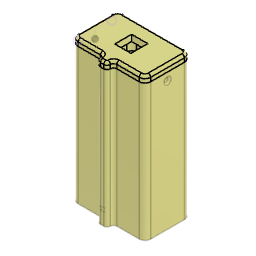
DelayPower Module Case (Autodesk Fusion 360 design; units mm, degrees)
Autodesk Fusion 360 part; units mm, degrees
sketch "Footprint" plane through (0, 0, 0) normal (0, 0, 1) x (1, 0, 0) in component "Case"
  line L0 (-12.76, 11.28) -> (12.76, 11.28)
  line L1 (15.18, 8.86) -> (15.18, -8.86)
  line L2 (12.76, -11.28) -> (-12.76, -11.28)
  line L3 (-15.18, -8.86) -> (-15.18, 8.86)
  arc A0 (-12.76, 11.28) -> (-15.18, 8.86) centre (-12.76, 8.86) ccw
  arc A1 (-15.18, -8.86) -> (-12.76, -11.28) centre (-12.76, -8.86) ccw
  arc A2 (12.76, -11.28) -> (15.18, -8.86) centre (12.76, -8.86) ccw
  arc A3 (15.18, 8.86) -> (12.76, 11.28) centre (12.76, 8.86) ccw
  line L4 (-7.205, 3.285) -> (-5.445, 3.285)
  line L5 (-5.445, 3.285) -> (-5.445, -3.285)
  line L6 (-5.445, -3.285) -> (-7.205, -3.285)
  line L7 (-7.205, -3.285) -> (-7.205, 3.285)
  line L8 (0, -11.28) -> (0, 11.28) construction
  line L9 (0, 0) -> (-5.445, 0) construction
  line L10 (7.205, -3.285) -> (7.205, 3.285)
  line L11 (5.445, 3.285) -> (5.445, -3.285)
  line L12 (7.205, 3.285) -> (5.445, 3.285)
  line L13 (5.445, -3.285) -> (7.205, -3.285)
  arc A4 (-18.6, 13.78) -> (-22.1, 10.28) centre (-18.6, 10.28) ccw
  line L14 (-22.1, -10.28) -> (-22.1, 10.28)
  arc A5 (-22.1, -10.28) -> (-18.6, -13.78) centre (-18.6, -10.28) ccw
  line L15 (-5, -13.78) -> (-18.6, -13.78)
  arc A6 (18.6, -13.78) -> (22.1, -10.28) centre (18.6, -10.28) ccw
  line L16 (22.1, 10.28) -> (22.1, -10.28)
  arc A7 (22.1, 10.28) -> (18.6, 13.78) centre (18.6, 10.28) ccw
  line L17 (-18.6, 13.78) -> (18.6, 13.78)
  line L18 (3, -15.7772) -> (3, -15.7772)
  line L19 (1, -17.78) -> (-1, -17.78)
  line L20 (-3, -15.7772) -> (-3, -15.7772)
  line L21 (1.8, -13.78) -> (1.8, -16.58)
  line L22 (1.8, -16.58) -> (-1.8, -16.58)
  line L23 (-1.8, -16.58) -> (-1.8, -13.78)
  arc A8 (-3, -15.7772) -> (-5, -13.78) centre (-5, -15.78) ccw
  line L24 (18.6, -13.78) -> (5, -13.78)
  arc A9 (5, -13.78) -> (3, -15.7772) centre (5, -15.78) ccw
  line L25 (1.8, -13.78) -> (-1.8, -13.78)
  line L26 (0, -11.28) -> (0, -13.78) construction
  arc A10 (-3, -15.7772) -> (-1, -17.78) centre (-1, -15.78) ccw
  arc A11 (1, -17.78) -> (3, -15.7772) centre (1, -15.78) ccw
  line L27 (19.6, -11.28) -> (19.6, 11.28)
  line L28 (-19.6, 11.28) -> (-19.6, -11.28)
  line L29 (-12.76, -11.28) -> (-19.6, -11.28)
  line L30 (12.76, -11.28) -> (19.6, -11.28)
  line L31 (12.76, 11.28) -> (19.6, 11.28)
  line L32 (-12.76, 11.28) -> (-19.6, 11.28)
  point P0 (5.445, 0)
  dimension "d1" = 2.42
  dimension "d2" = 2.42
  dimension "d3" = 2.42
  dimension "d4" = 2.42
  dimension "d5" = 30.36
  dimension "d6" = 22.56
  dimension "d7" = 1.76
  dimension "d8" = 6.57
  dimension "d9" = 5.445
  dimension "d15" = 1.2
  dimension "d16" = 2
  dimension "d17" = 2
  dimension "d23" = 2
  dimension "d24" = 2
  dimension "d25" = 1.2
  dimension "d26" = 1.2
  dimension "d27" = 4
  dimension "d28" = 6
  dimension "d76" = 3.5
  dimension "d77" = 3.5
  dimension "d78" = 3.5
  dimension "d79" = 3.5
  dimension "d80" = 39.2
  dimension "d81" = 2.5
  dimension "d82" = 2.5
  dimension "d83" = 2.5
  constraint horizontal L0
  constraint vertical L1
  constraint horizontal L2
  constraint vertical L3
  constraint tangent L0 A0
  constraint tangent L3 A0
  constraint tangent L2 A1
  constraint tangent L3 A1
  constraint tangent L1 A2
  constraint tangent L2 A2
  constraint tangent L0 A3
  constraint tangent L1 A3
  constraint horizontal L4
  constraint vertical L5
  constraint horizontal L6
  constraint vertical L7
  constraint midpoint L2 L8.start
  constraint midpoint L0 L8.end
  constraint midpoint L9.start L8
  constraint coincident L9.start origin
  constraint midpoint L5 L9.end
  constraint horizontal L9
  constraint symmetric L4.start L8 L10.end
  constraint symmetric L4.end L8 L11.start
  constraint symmetric L5.end L8 L11.end
  constraint symmetric L6.end L8 L10.start
  constraint symmetric L8 L9.end P0
  constraint horizontal L19
  constraint coincident L15 L21.start
  constraint perpendicular L15 L21
  constraint coincident L15 L23.end
  constraint perpendicular L22 L23
  constraint parallel L3 L14
  constraint parallel L2 L15
  constraint parallel L1 L16
  constraint parallel L0 L17
  constraint tangent A4 L17
  constraint tangent A4 L14
  constraint tangent A7 L17
  constraint tangent L14 A5
  constraint tangent A5 L15
  constraint tangent L16 A7
  constraint tangent L15 A6
  constraint tangent A6 L16
  constraint coincident A6.start L15
  constraint tangent L15 A8
  constraint tangent A6 L24
  constraint tangent L24 A9
  constraint midpoint L25 L26.end
  constraint perpendicular L25 L26
  constraint tangent L19 A10
  constraint tangent L19 A11
  constraint equal L15 L24
  constraint vertical L27
  constraint vertical L28
  constraint perpendicular L28 L29
  constraint perpendicular L27 L30
  constraint perpendicular L28 L32
  constraint perpendicular L27 L31
  constraint equal L29 L30
  measures "d1" radius of A0
  measures "d2" radius of A1
  measures "d3" radius of A2
  measures "d4" radius of A3
  measures "d5" distance of L1 L3
  measures "d6" distance of L0 L2
  measures "d7" distance of L4.start L4.end
  measures "d8" distance of L4.start L6.end
  measures "d9" distance of L9.start L9.end
  measures "d15" distance of L19 L22
  measures "d16" radius of A8
  measures "d17" radius of A9
  measures "d23" radius of A10
  measures "d24" radius of A11
  measures "d25" distance of L21 L18.start
  measures "d26" distance of L23 L20.start
  measures "d27" distance of L19 L24
  measures "d28" distance of L20.start L18.start
  measures "d76" radius of A5
  measures "d77" radius of A6
  measures "d78" radius of A7
  measures "d79" radius of A4
  measures "d80" distance of L27 L28
  measures "d81" distance of L14 L28
  measures "d82" distance of L2 L15
  measures "d83" distance of L0 L17
extrude "Extrude1" add sketch "Footprint" along normal blind 1.1 contours L0 L1 L2 L3 A0 A1 A2 A3 | L3 A0 A1 L28 L29 L32 | L1 A2 A3 L27 L30 L31 | A4 L14 A5 L15 A6 L16 A7 L17 L19 A8 L24 A9 A10 A11 | L21 L22 L23 L25 makes body 1 in component "Case"
extrude "Extrude2" add sketch "Footprint" along normal blind 81.8 from surface at 1.1 contours A4 L14 A5 L15 A6 L16 A7 L17 L19 A8 L24 A9 A10 A11 bodies 1 in component "Case"
sketch "WireCutouts" plane through (0, -13.78, 0) normal (0, -1, 0) x (1, 0, 0) in component "Case"
  line L0 (-1.8, 1.1) -> (1.8, 1.1)
  line L1 (1.8, 1.1) -> (1.8, 82.9)
  line L2 (1.8, 82.9) -> (-1.8, 82.9)
  line L3 (-1.8, 82.9) -> (-1.8, 1.1)
  line L4 (1.8, 67.9) -> (-1.8, 67.9)
  line L5 (1.8, 10.1) -> (-1.8, 10.1)
  line L6 (1.8, 7.1) -> (-1.8, 7.1)
  dimension "d29" = 15
  dimension "d30" = 3
  dimension "d31" = 6
  constraint coincident L1 L4.start
  constraint coincident L3 L4.end
  constraint perpendicular L3 L4
  constraint coincident L1 L5.start
  constraint coincident L3 L5.end
  constraint perpendicular L3 L5
  constraint coincident L1 L6.start
  constraint coincident L3 L6.end
  constraint perpendicular L3 L6
  measures "d29" distance of L2 L4
  measures "d30" distance of L5 L6
  measures "d31" distance of L0 L6
extrude "Extrude3" cut sketch "WireCutouts" against normal up to surface (2.5 mm away) contours L1 L2 L3 L4 bodies 1 in component "Case"
extrude "Extrude4" cut sketch "WireCutouts" along normal up to surface (1.2 mm away) draft -25 from surface at 2.8 contours L1 L3 L5 L6 bodies 1 in component "Case"
chamfer "Chamfer1" distance 0.5 angle 45 4 edges at (0, -13.78, 67.9) (-1.8, -13.93, 82.9) (0, -16.58, 82.9) (1.8, -13.93, 82.9) on bodies 1 in component "Case"
sketch "Profile" plane through (0, 0, 0) normal (0, 0, 1) x (1, 0, 0) in component "Plug Retainer"
  line L0 (-19.6, 11.28) -> (-19.6, -11.28)
  line L1 (-12.76, 11.28) -> (-19.6, 11.28)
  line L2 (-12.76, 11.28) -> (12.76, 11.28)
  line L3 (12.76, 11.28) -> (19.6, 11.28)
  line L4 (19.6, -11.28) -> (19.6, 11.28)
  line L5 (12.76, -11.28) -> (19.6, -11.28)
  line L6 (12.76, -11.28) -> (-12.76, -11.28)
  line L7 (-12.76, -11.28) -> (-19.6, -11.28)
  line L8 (-12.76, -11.125) -> (-19.445, -11.125)
  line L9 (-19.445, 11.125) -> (-19.445, -11.125)
  line L10 (-12.76, 11.125) -> (-19.445, 11.125)
  line L11 (-12.76, 11.125) -> (12.76, 11.125)
  line L12 (12.76, 11.125) -> (19.445, 11.125)
  line L13 (19.445, -11.125) -> (19.445, 11.125)
  line L14 (12.76, -11.125) -> (19.445, -11.125)
  line L15 (12.76, -11.125) -> (-12.76, -11.125)
  line L16 (-12.76, 8.86) -> (12.76, 8.86)
  line L17 (12.76, 8.86) -> (12.76, -8.86)
  line L18 (12.76, -8.86) -> (-12.76, -8.86)
  line L19 (-12.76, -8.86) -> (-12.76, 8.86)
  line L20 (-17.6, 10.08) -> (17.6, 10.08)
  line L21 (17.6, 10.08) -> (17.6, -10.08)
  line L22 (17.6, -10.08) -> (-17.6, -10.08)
  line L23 (-17.6, -10.08) -> (-17.6, 10.08)
  point P0 (-12.76, 8.86)
  point P1 (-12.76, -8.86)
  point P2 (12.76, -8.86)
  point P3 (12.76, 8.86)
  dimension "d84" = 0.155
  dimension "d85" = 2
  dimension "d86" = 2
  dimension "d87" = 1.2
  dimension "d88" = 1.2
  constraint horizontal L16
  constraint vertical L17
  constraint horizontal L18
  constraint vertical L19
  constraint coincident P2 L17.end
  constraint coincident P0 L16.start
  constraint horizontal L20
  constraint vertical L21
  constraint horizontal L22
  constraint vertical L23
  measures "d85" distance of L4 L21
  measures "d86" distance of L0 L23
  measures "d87" distance of L6 L22
  measures "d88" distance of L2 L20
extrude "Extrude1'" add sketch "Profile" along normal blind 3 from surface at 4.9 separate body contours L8 L9 L10 L11 L12 L13 L14 L15 | L20 L21 L22 L23 makes body 2 in component "Plug Retainer"
extrude "Extrude3'" add sketch "Profile" along normal up to surface (67 mm away) from surface at 7.9 contours L8 L9 L10 L11 L12 L13 L14 L15 bodies 2 in component "Plug Retainer"
extrude "Extrude2'" cut sketch "WireCutouts" against normal up to surface (3.7 mm away) contours L1 L2 L3 L4 bodies 2 in component "Plug Retainer"
sketch "Footprint (2)" plane through (0, 0, 0) normal (0, 0, 1) x (1, 0, 0) in component "Lid"
  arc A0 (-3, -15.7772) -> (-5, -13.78) centre (-5, -15.78) ccw
  line L0 (-5, -13.78) -> (-18.6, -13.78)
  arc A1 (-22.1, -10.28) -> (-18.6, -13.78) centre (-18.6, -10.28) ccw
  line L1 (-22.1, -10.28) -> (-22.1, 10.28)
  arc A2 (-18.6, 13.78) -> (-22.1, 10.28) centre (-18.6, 10.28) ccw
  line L2 (-18.6, 13.78) -> (18.6, 13.78)
  arc A3 (22.1, 10.28) -> (18.6, 13.78) centre (18.6, 10.28) ccw
  arc A4 (18.6, -13.78) -> (22.1, -10.28) centre (18.6, -10.28) ccw
  line L3 (18.6, -13.78) -> (5, -13.78)
  arc A5 (5, -13.78) -> (3, -15.7772) centre (5, -15.78) ccw
  line L4 (22.1, 10.28) -> (22.1, -10.28)
  arc A6 (1, -17.78) -> (3, -15.7772) centre (1, -15.78) ccw
  arc A7 (-3, -15.7772) -> (-1, -17.78) centre (-1, -15.78) ccw
  line L5 (1, -17.78) -> (-1, -17.78)
  line L6 (-5.905, 9.105) -> (5.905, 9.105)
  line L7 (8.905, 6.105) -> (8.905, -6.105)
  line L8 (5.905, -9.105) -> (-5.905, -9.105)
  line L9 (-8.905, -6.105) -> (-8.905, 6.105)
  line L10 (15.025, 0) -> (8.905, 0) construction
  line L11 (0, 9.105) -> (0, 11.125) construction
  arc A8 (-5.905, 9.105) -> (-8.905, 6.105) centre (-5.905, 6.105) ccw
  arc A9 (-8.905, -6.105) -> (-5.905, -9.105) centre (-5.905, -6.105) ccw
  arc A10 (5.905, -9.105) -> (8.905, -6.105) centre (5.905, -6.105) ccw
  arc A11 (8.905, 6.105) -> (5.905, 9.105) centre (5.905, 6.105) ccw
  line L12 (-4.905, 5.105) -> (4.905, 5.105)
  line L13 (4.905, 5.105) -> (4.905, -5.105)
  line L14 (4.905, -5.105) -> (-4.905, -5.105)
  line L15 (-4.905, -5.105) -> (-4.905, 5.105)
  line L16 (8.905, 0) -> (4.905, 0) construction
  line L17 (0, 9.105) -> (0, 5.105) construction
  line L18 (-19.445, 11.125) -> (-19.445, -11.125)
  line L19 (-12.76, 11.125) -> (-19.445, 11.125)
  line L20 (-12.76, 11.125) -> (12.76, 11.125)
  line L21 (12.76, 11.125) -> (19.445, 11.125)
  line L22 (19.445, -11.125) -> (19.445, 11.125)
  line L23 (12.76, -11.125) -> (19.445, -11.125)
  line L24 (12.76, -11.125) -> (-12.76, -11.125)
  line L25 (-12.76, -11.125) -> (-19.445, -11.125)
  dimension "d14" = 1.2
  dimension "d71" = 3
  dimension "d72" = 9.81
  dimension "d73" = 10.21
  dimension "d74" = 4
  dimension "d75" = 4
  constraint horizontal L6
  constraint vertical L7
  constraint horizontal L8
  constraint vertical L9
  constraint vertical L11
  constraint horizontal L10
  constraint coincident L6 L11.start
  constraint tangent L6 A8
  constraint tangent L9 A8
  constraint tangent L8 A9
  constraint tangent L9 A9
  constraint equal A8 A9
  constraint coincident L7 L10.end
  constraint tangent L7 A10
  constraint tangent L8 A10
  constraint equal A8 A10
  constraint tangent L6 A11
  constraint tangent L7 A11
  constraint equal A8 A11
  constraint midpoint L7 L10.end
  constraint midpoint L6 L11.start
  constraint horizontal L12
  constraint vertical L13
  constraint horizontal L14
  constraint vertical L15
  constraint midpoint L13 L16.end
  constraint midpoint L12 L17.end
  constraint vertical L17
  constraint horizontal L16
  constraint midpoint L11.end L20
  measures "d71" radius of A8
  measures "d72" distance of L13.end L14.end
  measures "d73" distance of L12.end L13.end
  measures "d74" distance of L11.start L17.end
  measures "d75" distance of L9 L15
extrude "Extrude4'" add sketch "Footprint (2)" along normal up to surface (8 mm away) from surface at 75.055 separate body contours L18 L19 L20 L21 L22 L23 L24 L25 makes body 3 in component "Lid"
extrude "Extrude5" add sketch "Footprint (2)" along normal blind 3.8 from surface at 83.055 contours A0 L0 A1 L1 A2 L2 A3 A4 L3 A5 L4 A6 A7 L5 | L6 L7 L8 L9 A8 A9 A10 A11 | L18 L19 L20 L21 L22 L23 L24 L25 bodies 3 in component "Lid"
fillet "Fillet2" radius 1.5 14 edges at (3.5868, -14.3648, 86.855) (11.8, -13.78, 86.855) (21.0749, -12.7549, 86.855) (22.1, 0, 86.855) (21.0749, 12.7549, 86.855) (0, 13.78, 86.855) (-21.0749, 12.7549, 86.855) (-22.1, 0, 86.855) (-21.0749, -12.7549, 86.855) (-11.8, -13.78, 86.855) (-3.5868, -14.3648, 86.855) (-2.4152, -17.1932, 86.855) (0, -17.78, 86.855) (2.4152, -17.1932, 86.855) on bodies 3 in component "Lid"
chamfer "Chamfer2" distance 0.9 angle 45 5 edges at (19.6, 0, 82.9) (0, 11.28, 82.9) (-19.6, 0, 82.9) (-10.95, -11.28, 82.9) (10.95, -11.28, 82.9) on bodies 1 in component "Case"
fillet "Fillet1" radius 2 4 edges at (-20.05, 11.73, 82.45) (20.05, -11.73, 82.45) (20.05, 11.73, 82.45) (-20.05, -11.73, 82.45) on bodies 1 in component "Case"
sketch "Screws" plane through (-22.1, 0, 0) normal (-1, 0, 0) x (0, -1, 0)
  line L0 (-10.28, 82.9) -> (10.28, 82.9)
  circle A0 centre (0, 78.4) radius 1.22
  line L1 (0, 78.4) -> (0, 82.9) construction
  dimension "d99" = 2.44
  dimension "d107" = 4.5
  constraint coincident A0.centre L1.start
  constraint midpoint L0 L1.end
  constraint perpendicular L0 L1
  measures "d99" diameter of A0
  measures "d107" distance of A0.centre L1.end
extrude "Extrude5'" cut sketch "Screws" against normal up to surface (44.2 mm away) bodies 1 in component "Case"
chamfer "Chamfer3" distance 1 angle 45 2 edges at (-22.1, 1.1374, 78.8412) (22.1, 1.1374, 77.9588) on bodies 1 in component "Case"
extrude "Extrude6" cut sketch "Screws" against normal up to surface (38.89 mm away) from surface at -2.655 bodies 3 in component "Lid"
component "Case" placed x (1, 0, 0) y (0, 1, 0) z (0, 0, 1) at (0, 0, 0)
component "Plug Retainer" placed x (1, 0, 0) y (0, 1, 0) z (0, 0, 1) at (0, 0, 0)
component "Lid" placed x (1, 0, 0) y (0, 1, 0) z (0, 0, 1) at (0, 0, 0)
equation "d2 = d1"
equation "d3 = d1"
equation "d4 = d1"
equation "d5 = 30.05 mm + 2 * Tolerance_Tight"
equation "d6 = 22.25 mm + 2 * Tolerance_Tight"
equation "d7 = 1.45 mm + 2 * Tolerance_Tight"
equation "d8 = 6.26 mm + 2 * Tolerance_Tight"
equation "d9 = 5.6 mm - Tolerance_Tight"
equation "d15 = d26"
equation "d17 = d16"
equation "d23 = d16"
equation "d24 = d16"
equation "d25 = d26"
equation "Tolerance = 0.17 mm"
equation "Tolerance_Tight = 0.155 mm"
equation "Tolerance_PressFitLight = 0.12 mm"
equation "d63 = Tolerance_Tight"
equation "d64 = Tolerance_Tight"
equation "d75 = d74"
equation "d77 = d76"
equation "d78 = d76"
equation "d79 = d76"
equation "d82 = d81"
equation "d83 = d81"
equation "d84 = Tolerance_Tight"
equation "d85 = d86"
equation "d87 = d88"
equation "Screw_Diameter = 2.2 mm"
equation "Screw_Length = 11.3 mm"
equation "Screw_ChamferSize = 1 mm" comment "The depth of the chamfer is 1 mm, diameter is 4.2mm"
equation "NutInnerCircle_Radius = 2.495 mm"
equation "d99 = Screw_Diameter + 2 * Tolerance_PressFitLight"
equation "d103 = Screw_ChamferSize"
